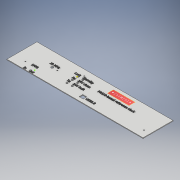
# Autodesk Inventor part: Panel
Saved by Autodesk Inventor 2018.2 (Build 222227000, 227)
## iProperties
Created: 2018-05-24
Part Number: Panel
Material: Generic
Document SubType Name: Modeling
Designer: ShifT
Density: 1 g/cm^3
Appearance: Default
Author: ShifT
Autodesk Inventor part; units mm, degrees
(part 1 of 3)
ref_plane "YZ Plane" through (0, 0, 0) normal (1, 0, 0) x (0, 1, 0)
ref_plane "XZ Plane" through (0, 0, 0) normal (0, 1, 0) x (-1, 0, 0)
ref_plane "XY Plane" through (0, 0, 0) normal (0, 0, 1) x (1, 0, 0)
sketch "Cutouts" plane through (0, 0, 0) normal (0, 0, 1) x (1, 0, 0)
  line L0 (-147.3514, 29.5026) -> (251.6486, 29.5026)
  line L1 (251.6486, 29.5026) -> (251.6486, -58.4974)
  line L2 (251.6486, -58.4974) -> (-147.3514, -58.4974)
  line L3 (-147.3514, -58.4974) -> (-147.3514, 29.5026)
  circle A0 centre (1, 0) radius 2.5548
  circle A1 centre (16.329, 0) radius 2.5548
  circle A2 centre (1, -15.329) radius 2.5548
  circle A3 centre (1, -30.6581) radius 2.5548
  circle A4 centre (16.329, -15.329) radius 2.5548
  circle A5 centre (16.329, -30.6581) radius 2.5548
  line L4 (53.6111, -37.1691) -> (65.6111, -37.1691)
  line L5 (65.6111, -37.1691) -> (65.6111, -47.8691)
  line L6 (65.6111, -47.8691) -> (53.6111, -47.8691)
  line L7 (53.6111, -47.8691) -> (53.6111, -37.1691)
  arc A6 (217.5748, -12.7276) -> (217.5951, -14.9758) centre (207.3252, -13.9442) ccw
  line L8 (217.6303, -12.7276) -> (218.5501, -12.7276)
  line L9 (218.5501, -12.7276) -> (218.5501, -14.9758)
  line L10 (218.5501, -14.9758) -> (217.5589, -14.9758)
  line L11 (207.3252, -13.9442) -> (219.4574, -13.9442) construction
  arc A7 (-61.8557, -10.0731) -> (-58.5401, -10.0731) centre (-60.1979, -12.8975) ccw
  line L12 (-61.8557, -10.0731) -> (-58.5401, -10.0731)
  arc A8 (-99.5904, -43.7211) -> (-96.2748, -43.7211) centre (-97.9326, -46.5455) ccw
  line L13 (-99.5904, -43.7211) -> (-96.2748, -43.7211)
  arc A9 (-80.2876, -43.5409) -> (-76.972, -43.5409) centre (-78.6298, -46.3653) ccw
  line L14 (-80.2876, -43.5409) -> (-76.972, -43.5409)
  circle A10 centre (9, 12) radius 1.5
  circle A11 centre (234, -38) radius 1.5
  circle A12 centre (-44.6116, -13.1835) radius 1.5
  circle A13 centre (-114.7272, -37.1581) radius 1.5
  point P0 (0, 0)
  dimension "d29" = 88
  dimension "d34" = 12
  dimension "d35" = 10.7
  dimension "d38" = 399
  dimension "d59" = 3.275
  dimension "d60" = 3.275
  dimension "d61" = 3.275
  constraints: 30 end point, 14 centre point, 8 point on circle, 5 horizontal, 5 parallel, 2 perpendicular, 2 point on line
  measures "d29" distance of L0.end L1.end
  measures "d34" distance of L4.start L4.end
  measures "d35" distance of L4.end L5.end
  measures "d38" distance of L0.start L0.end
  measures "d59" radius of A7
  measures "d60" radius of A9
  measures "d61" radius of A8
sketch "Text" plane through (0, 0, 0) normal (0, 0, 1) x (1, 0, 0)
  line L0 (-5.0504, -5.8552) -> (4.5125, -5.8552) construction
  line L1 (4.5125, -5.8552) -> (4.5125, -12.089) construction
  line L2 (4.5125, -12.089) -> (-5.0504, -12.089) construction
  line L3 (-5.0504, -12.089) -> (-5.0504, -5.8552) construction
  line L4 (-5.6331, -20.25) -> (3.6166, -20.25) construction
  line L5 (3.6166, -20.25) -> (3.6166, -26.4838) construction
  line L6 (3.6166, -26.4838) -> (-5.6331, -26.4838) construction
  line L7 (-5.6331, -26.4838) -> (-5.6331, -20.25) construction
  line L8 (11.6752, 9.4343) -> (42.3442, 9.4343) construction
  line L9 (42.3442, 9.4343) -> (42.3442, 1.2001) construction
  line L10 (42.3442, 1.2001) -> (11.6752, 1.2001) construction
  line L11 (11.6752, 1.2001) -> (11.6752, 9.4343) construction
  line L12 (11.9113, -5.446) -> (48.7686, -5.446) construction
  line L13 (48.7686, -5.446) -> (48.7686, -12.089) construction
  line L14 (48.7686, -12.089) -> (11.9113, -12.089) construction
  line L15 (11.9113, -12.089) -> (11.9113, -5.446) construction
  line L16 (12.7825, -20.3944) -> (46.5936, -20.3944) construction
  line L17 (46.5936, -20.3944) -> (46.5936, -27.0374) construction
  line L18 (46.5936, -27.0374) -> (12.7825, -27.0374) construction
  line L19 (12.7825, -27.0374) -> (12.7825, -20.3944) construction
  line L20 (-12.4705, 9.78) -> (4.6093, 9.78) construction
  line L21 (4.6093, 9.78) -> (4.6093, 1.0076) construction
  line L22 (4.6093, 1.0076) -> (-12.4705, 1.0076) construction
  line L23 (-12.4705, 1.0076) -> (-12.4705, 9.78) construction
  line L24 (-74.187, -1.4436) -> (-45.9479, -1.4436) construction
  line L25 (-45.9479, -1.4436) -> (-45.9479, -7.9351) construction
  line L26 (-45.9479, -7.9351) -> (-74.187, -7.9351) construction
  line L27 (-74.187, -7.9351) -> (-74.187, -1.4436) construction
  line L28 (-85.9199, -50.8606) -> (-71.5682, -50.8606) construction
  line L29 (-71.5682, -50.8606) -> (-71.5682, -58.0237) construction
  line L30 (-71.5682, -58.0237) -> (-85.9199, -58.0237) construction
  line L31 (-85.9199, -58.0237) -> (-85.9199, -50.8606) construction
  line L32 (-97.5821, -32.5156) -> (-80.0066, -32.5156) construction
  line L33 (-80.0066, -32.5156) -> (-80.0066, -38.9717) construction
  line L34 (-80.0066, -38.9717) -> (-97.5821, -38.9717) construction
  line L35 (-97.5821, -38.9717) -> (-97.5821, -32.5156) construction
  line L36 (69.2256, -39.9947) -> (96.6261, -39.9947) construction
  line L37 (96.6261, -39.9947) -> (96.6261, -46.4912) construction
  line L38 (96.6261, -46.4912) -> (69.2256, -46.4912) construction
  line L39 (69.2256, -46.4912) -> (69.2256, -39.9947) construction
  line L40 (86.2036, 20.2511) -> (149.6463, 20.2511) construction
  line L41 (149.6463, 20.2511) -> (149.6463, 2.3892) construction
  line L42 (149.6463, 2.3892) -> (86.2036, 2.3892) construction
  line L43 (86.2036, 2.3892) -> (86.2036, 20.2511) construction
  line L44 (67.8583, -2.9005) -> (181.6324, -2.9005) construction
  line L45 (181.6324, -2.9005) -> (181.6324, -16.7416) construction
  line L46 (181.6324, -16.7416) -> (67.8583, -16.7416) construction
  line L47 (67.8583, -16.7416) -> (67.8583, -2.9005) construction
  line L48 (-102.0131, -51.196) -> (-93.5064, -51.196) construction
  line L49 (-93.5064, -51.196) -> (-93.5064, -57.9236) construction
  line L50 (-93.5064, -57.9236) -> (-102.0131, -57.9236) construction
  line L51 (-102.0131, -57.9236) -> (-102.0131, -51.196) construction
  line L52 (-99.2695, -57.296) -> (-101.6324, -57.296)
  line L53 (-101.6324, -57.296) -> (-101.6324, -56.6731)
  line L54 (-101.6324, -56.6731) -> (-100.8563, -56.6731)
  line L55 (-100.8563, -56.6731) -> (-100.8563, -51.8188)
  line L56 (-100.8563, -51.8188) -> (-101.6324, -51.8188)
  line L57 (-101.6324, -51.8188) -> (-101.6324, -51.196)
  line L58 (-101.6324, -51.196) -> (-99.2695, -51.196)
  line L59 (-99.2695, -51.196) -> (-99.2695, -51.8188)
  line L60 (-99.2695, -51.8188) -> (-100.0456, -51.8188)
  line L61 (-100.0456, -51.8188) -> (-100.0456, -56.6731)
  line L62 (-100.0456, -56.6731) -> (-99.2695, -56.6731)
  line L63 (-99.2695, -56.6731) -> (-99.2695, -57.296)
  line L64 (-94.7316, -57.296) -> (-95.5028, -57.296)
  line L65 (-95.5028, -57.296) -> (-95.5028, -54.6859)
  spline S0 degree 2 poles (-95.5028, -54.6859) (-95.5028, -54.3696) (-95.5621, -53.8258) (-95.6511, -53.6627) knots 0 0 0 1 2 2 2
  spline S1 degree 2 poles (-95.6511, -53.6627) (-95.745, -53.4897) (-96.0811, -53.3216) (-96.3678, -53.3216) knots 0 0 0 1 2 2 2
  spline S2 degree 2 poles (-96.3678, -53.3216) (-96.6546, -53.3216) (-97.2626, -53.6281) (-97.5542, -53.8752) knots 0 0 0 1 2 2 2
  line L66 (-97.5542, -53.8752) -> (-97.5542, -57.296)
  line L67 (-97.5542, -57.296) -> (-98.3254, -57.296)
  line L68 (-98.3254, -57.296) -> (-98.3254, -52.7185)
  line L69 (-98.3254, -52.7185) -> (-97.5542, -52.7185)
  line L70 (-97.5542, -52.7185) -> (-97.5542, -53.2277)
  spline S3 degree 2 poles (-97.5542, -53.2277) (-97.2082, -52.9162) (-96.5409, -52.59) (-96.1652, -52.59) knots 0 0 0 1 2 2 2
  spline S4 degree 2 poles (-96.1652, -52.59) (-95.4929, -52.59) (-94.7316, -53.4798) (-94.7316, -54.3251) knots 0 0 0 1 2 2 2
  line L71 (-94.7316, -54.3251) -> (-94.7316, -57.296)
  line L72 (-70.2867, -7.6672) -> (-73.2626, -7.6672)
  line L73 (-73.2626, -7.6672) -> (-73.2626, -7.0443)
  line L74 (-73.2626, -7.0443) -> (-72.1553, -7.0443)
  line L75 (-72.1553, -7.0443) -> (-72.1553, -2.9563)
  line L76 (-72.1553, -2.9563) -> (-73.2626, -2.9563)
  line L77 (-73.2626, -2.9563) -> (-73.2626, -2.3977)
  spline S5 degree 2 poles (-73.2626, -2.3977) (-72.6348, -2.3977) (-72.0416, -2.0418) (-72.002, -1.5474) knots 0 0 0 1 2 2 2
  line L78 (-72.002, -1.5474) -> (-71.3693, -1.5474)
  line L79 (-71.3693, -1.5474) -> (-71.3693, -7.0443)
  line L80 (-71.3693, -7.0443) -> (-70.2867, -7.0443)
  line L81 (-70.2867, -7.0443) -> (-70.2867, -7.6672)
  spline S6 degree 2 poles (-65.3682, -4.6172) (-65.3682, -6.2584) (-66.3222, -7.7957) (-67.3158, -7.7957) knots 0 0 0 1 2 2 2
  spline S7 degree 2 poles (-67.3158, -7.7957) (-68.3243, -7.7957) (-69.2684, -6.2287) (-69.2684, -4.6221) knots 0 0 0 1 2 2 2
  spline S8 degree 2 poles (-69.2684, -4.6221) (-69.2684, -2.9711) (-68.3144, -1.4436) (-67.3158, -1.4436) knots 0 0 0 1 2 2 2
  spline S9 degree 2 poles (-67.3158, -1.4436) (-66.3123, -1.4436) (-65.3682, -3.0255) (-65.3682, -4.6172) knots 0 0 0 1 2 2 2
  spline S10 degree 2 poles (-66.4161, -6.4759) (-66.2975, -6.1743) (-66.1986, -5.245) (-66.1986, -4.6172) knots 0 0 0 1 2 2 2
  spline S11 degree 2 poles (-66.1986, -4.6172) (-66.1986, -3.9894) (-66.2975, -3.065) (-66.4211, -2.7536) knots 0 0 0 1 2 2 2
  spline S12 degree 2 poles (-66.4211, -2.7536) (-66.5447, -2.4422) (-66.9747, -2.1208) (-67.3158, -2.1208) knots 0 0 0 1 2 2 2
  spline S13 degree 2 poles (-67.3158, -2.1208) (-67.6569, -2.1208) (-68.0969, -2.4422) (-68.2254, -2.7635) knots 0 0 0 1 2 2 2
  spline S14 degree 2 poles (-68.2254, -2.7635) (-68.349, -3.0749) (-68.4379, -4.024) (-68.4379, -4.6221) knots 0 0 0 1 2 2 2
  spline S15 degree 2 poles (-68.4379, -4.6221) (-68.4379, -5.2648) (-68.3589, -6.1249) (-68.2303, -6.461) knots 0 0 0 1 2 2 2
  spline S16 degree 2 poles (-68.2303, -6.461) (-68.1117, -6.7774) (-67.6717, -7.1185) (-67.3158, -7.1185) knots 0 0 0 1 2 2 2
  spline S17 degree 2 poles (-67.3158, -7.1185) (-66.9797, -7.1185) (-66.5397, -6.7972) (-66.4161, -6.4759) knots 0 0 0 1 2 2 2
  line L82 (-56.5642, -7.6672) -> (-57.3749, -7.6672)
  line L83 (-57.3749, -7.6672) -> (-57.3749, -2.4125)
  line L84 (-57.3749, -2.4125) -> (-58.9666, -5.9865)
  line L85 (-58.9666, -5.9865) -> (-59.461, -5.9865)
  line L86 (-59.461, -5.9865) -> (-61.0379, -2.4125)
  line L87 (-61.0379, -2.4125) -> (-61.0379, -7.6672)
  line L88 (-61.0379, -7.6672) -> (-61.7942, -7.6672)
  line L89 (-61.7942, -7.6672) -> (-61.7942, -1.5672)
  line L90 (-61.7942, -1.5672) -> (-60.6869, -1.5672)
  line L91 (-60.6869, -1.5672) -> (-59.1644, -4.9632)
  line L92 (-59.1644, -4.9632) -> (-57.6913, -1.5672)
  line L93 (-57.6913, -1.5672) -> (-56.5642, -1.5672)
  line L94 (-56.5642, -1.5672) -> (-56.5642, -7.6672)
  line L95 (-50.8992, -7.6672) -> (-51.7099, -7.6672)
  line L96 (-51.7099, -7.6672) -> (-51.7099, -4.6815)
  line L97 (-51.7099, -4.6815) -> (-54.5177, -4.6815)
  line L98 (-54.5177, -4.6815) -> (-54.5177, -7.6672)
  line L99 (-54.5177, -7.6672) -> (-55.3284, -7.6672)
  line L100 (-55.3284, -7.6672) -> (-55.3284, -1.5672)
  line L101 (-55.3284, -1.5672) -> (-54.5177, -1.5672)
  line L102 (-54.5177, -1.5672) -> (-54.5177, -3.9597)
  line L103 (-54.5177, -3.9597) -> (-51.7099, -3.9597)
  line L104 (-51.7099, -3.9597) -> (-51.7099, -1.5672)
  line L105 (-51.7099, -1.5672) -> (-50.8992, -1.5672)
  line L106 (-50.8992, -1.5672) -> (-50.8992, -7.6672)
  line L107 (-46.7172, -7.6672) -> (-50.0786, -7.6672)
  line L108 (-50.0786, -7.6672) -> (-50.0786, -7.0938)
  line L109 (-50.0786, -7.0938) -> (-47.6861, -3.7225)
  line L110 (-47.6861, -3.7225) -> (-49.9798, -3.7225)
  line L111 (-49.9798, -3.7225) -> (-49.9798, -3.0897)
  line L112 (-49.9798, -3.0897) -> (-46.7617, -3.0897)
  line L113 (-46.7617, -3.0897) -> (-46.7617, -3.6384)
  line L114 (-46.7617, -3.6384) -> (-49.1641, -7.0196)
  line L115 (-49.1641, -7.0196) -> (-46.7172, -7.0196)
  line L116 (-46.7172, -7.0196) -> (-46.7172, -7.6672)
  line L117 (-8.3182, 3.4081) -> (-11.8526, 3.4081)
  line L118 (-11.8526, 3.4081) -> (-11.8526, 9.5081)
  line L119 (-11.8526, 9.5081) -> (-11.0419, 9.5081)
  line L120 (-11.0419, 9.5081) -> (-11.0419, 4.1298)
  line L121 (-11.0419, 4.1298) -> (-8.3182, 4.1298)
  line L122 (-8.3182, 4.1298) -> (-8.3182, 3.4081)
  spline S18 degree 2 poles (-3.978, 5.6968) (-3.978, 4.5401) (-5.0902, 3.2796) (-6.0195, 3.2796) knots 0 0 0 1 2 2 2
  spline S19 degree 2 poles (-6.0195, 3.2796) (-6.9736, 3.2796) (-8.066, 4.5797) (-8.066, 5.6968) knots 0 0 0 1 2 2 2
  spline S20 degree 2 poles (-8.066, 5.6968) (-8.066, 6.8437) (-6.939, 8.1141) (-6.0195, 8.1141) knots 0 0 0 1 2 2 2
  spline S21 degree 2 poles (-6.0195, 8.1141) (-5.0902, 8.1141) (-3.978, 6.8486) (-3.978, 5.6968) knots 0 0 0 1 2 2 2
  spline S22 degree 2 poles (-4.7738, 5.6968) (-4.7738, 6.5866) (-5.4214, 7.4517) (-6.0195, 7.4517) knots 0 0 0 1 2 2 2
  spline S23 degree 2 poles (-6.0195, 7.4517) (-6.6177, 7.4517) (-7.2702, 6.5866) (-7.2702, 5.6968) knots 0 0 0 1 2 2 2
  spline S24 degree 2 poles (-7.2702, 5.6968) (-7.2702, 4.8318) (-6.6177, 3.942) (-6.0195, 3.942) knots 0 0 0 1 2 2 2
  spline S25 degree 2 poles (-6.0195, 3.942) (-5.4263, 3.942) (-4.7738, 4.8169) (-4.7738, 5.6968) knots 0 0 0 1 2 2 2
  spline S26 degree 2 poles (-1.3679, 3.3043) (-1.8425, 3.3043) (-2.6284, 3.596) (-2.9102, 3.8925) knots 0 0 0 1 2 2 2
  spline S27 degree 2 poles (-2.9102, 3.8925) (-3.192, 4.1842) (-3.5034, 5.0839) (-3.5034, 5.687) knots 0 0 0 1 2 2 2
  spline S28 degree 2 poles (-3.5034, 5.687) (-3.5034, 6.29) (-3.1821, 7.1699) (-2.9102, 7.4665) knots 0 0 0 1 2 2 2
  spline S29 degree 2 poles (-2.9102, 7.4665) (-2.6383, 7.7681) (-1.8326, 8.0894) (-1.3679, 8.0894) knots 0 0 0 1 2 2 2
  spline S30 degree 2 poles (-1.3679, 8.0894) (-0.9922, 8.0894) (-0.2903, 7.8768) (-0.0184, 7.7384) knots 0 0 0 1 2 2 2
  line L123 (-0.0184, 7.7384) -> (-0.0184, 6.8733)
  line L124 (-0.0184, 6.8733) -> (-0.0629, 6.8733)
  spline S31 degree 2 poles (-0.0629, 6.8733) (-0.1469, 6.9425) (-0.404, 7.1205) (-0.5869, 7.2144) knots 0 0 0 1 2 2 2
  spline S32 degree 2 poles (-0.5869, 7.2144) (-0.75, 7.2935) (-1.185, 7.4171) (-1.3827, 7.4171) knots 0 0 0 1 2 2 2
  spline S33 degree 2 poles (-1.3827, 7.4171) (-1.9809, 7.4171) (-2.7075, 6.5125) (-2.7075, 5.687) knots 0 0 0 1 2 2 2
  spline S34 degree 2 poles (-2.7075, 5.687) (-2.7075, 4.8812) (-2.0056, 3.9766) (-1.3827, 3.9766) knots 0 0 0 1 2 2 2
  spline S35 degree 2 poles (-1.3827, 3.9766) (-1.0071, 3.9766) (-0.3249, 4.288) (-0.0629, 4.5302) knots 0 0 0 1 2 2 2
  line L125 (-0.0629, 4.5302) -> (-0.0184, 4.5302)
  line L126 (-0.0184, 4.5302) -> (-0.0184, 3.6652)
  spline S36 degree 2 poles (-0.0184, 3.6652) (-0.1321, 3.6108) (-0.4781, 3.4575) (-0.6165, 3.4229) knots 0 0 0 1 2 2 2
  spline S37 degree 2 poles (-0.6165, 3.4229) (-0.8143, 3.3636) (-1.1257, 3.3043) (-1.3679, 3.3043) knots 0 0 0 1 2 2 2
  line L127 (4.475, 3.4081) -> (3.4617, 3.4081)
  line L128 (3.4617, 3.4081) -> (1.7612, 5.6177)
  line L129 (1.7612, 5.6177) -> (1.4547, 5.3212)
  line L130 (1.4547, 5.3212) -> (1.4547, 3.4081)
  line L131 (1.4547, 3.4081) -> (0.6835, 3.4081)
  line L132 (0.6835, 3.4081) -> (0.6835, 9.78)
  line L133 (0.6835, 9.78) -> (1.4547, 9.78)
  line L134 (1.4547, 9.78) -> (1.4547, 6.0528)
  line L135 (1.4547, 6.0528) -> (3.2639, 7.9856)
  line L136 (3.2639, 7.9856) -> (4.2229, 7.9856)
  line L137 (4.2229, 7.9856) -> (2.3445, 6.0725)
  line L138 (2.3445, 6.0725) -> (4.475, 3.4081)
  spline S38 degree 2 poles (-80.9865, -51.6861) (-80.6405, -52.0914) (-80.2549, -53.2778) (-80.2549, -54.0391) knots 0 0 0 1 2 2 2
  spline S39 degree 2 poles (-80.2549, -54.0391) (-80.2549, -54.7806) (-80.6306, -55.9818) (-80.9865, -56.3871) knots 0 0 0 1 2 2 2
  spline S40 degree 2 poles (-80.9865, -56.3871) (-81.3622, -56.8123) (-82.3558, -57.2176) (-82.954, -57.2176) knots 0 0 0 1 2 2 2
  spline S41 degree 2 poles (-82.954, -57.2176) (-83.5719, -57.2176) (-84.5605, -56.7974) (-84.9214, -56.3871) knots 0 0 0 1 2 2 2
  spline S42 degree 2 poles (-84.9214, -56.3871) (-85.2724, -55.9818) (-85.648, -54.7905) (-85.648, -54.0391) knots 0 0 0 1 2 2 2
  spline S43 degree 2 poles (-85.648, -54.0391) (-85.648, -53.2729) (-85.2674, -52.1063) (-84.9164, -51.6861) knots 0 0 0 1 2 2 2
  spline S44 degree 2 poles (-84.9164, -51.6861) (-84.5605, -51.2807) (-83.5669, -50.8606) (-82.954, -50.8606) knots 0 0 0 1 2 2 2
  spline S45 degree 2 poles (-82.954, -50.8606) (-82.3311, -50.8606) (-81.3326, -51.2956) (-80.9865, -51.6861) knots 0 0 0 1 2 2 2
  spline S46 degree 2 poles (-81.1002, -54.0391) (-81.1002, -53.436) (-81.3622, -52.5017) (-81.5995, -52.1952) knots 0 0 0 1 2 2 2
  spline S47 degree 2 poles (-81.5995, -52.1952) (-81.8417, -51.8789) (-82.5239, -51.5625) (-82.949, -51.5625) knots 0 0 0 1 2 2 2
  spline S48 degree 2 poles (-82.949, -51.5625) (-83.389, -51.5625) (-84.0514, -51.869) (-84.3035, -52.1952) knots 0 0 0 1 2 2 2
  spline S49 degree 2 poles (-84.3035, -52.1952) (-84.5457, -52.5067) (-84.8027, -53.4459) (-84.8027, -54.0391) knots 0 0 0 1 2 2 2
  spline S50 degree 2 poles (-84.8027, -54.0391) (-84.8027, -55.2403) (-83.7943, -56.5157) (-82.949, -56.5157) knots 0 0 0 1 2 2 2
  spline S51 degree 2 poles (-82.949, -56.5157) (-82.1037, -56.5157) (-81.1002, -55.2403) (-81.1002, -54.0391) knots 0 0 0 1 2 2 2
  line L139 (-75.8653, -57.0891) -> (-76.6365, -57.0891)
  line L140 (-76.6365, -57.0891) -> (-76.6365, -56.5849)
  spline S52 degree 2 poles (-76.6365, -56.5849) (-76.9924, -56.8963) (-77.6301, -57.2176) (-78.0255, -57.2176) knots 0 0 0 1 2 2 2
  spline S53 degree 2 poles (-78.0255, -57.2176) (-78.3221, -57.2176) (-78.851, -57.0199) (-79.0438, -56.8073) knots 0 0 0 1 2 2 2
  spline S54 degree 2 poles (-79.0438, -56.8073) (-79.2416, -56.5948) (-79.4591, -55.9472) (-79.4591, -55.4825) knots 0 0 0 1 2 2 2
  line L141 (-79.4591, -55.4825) -> (-79.4591, -52.5116)
  line L142 (-79.4591, -52.5116) -> (-78.6879, -52.5116)
  line L143 (-78.6879, -52.5116) -> (-78.6879, -55.1217)
  spline S55 degree 2 poles (-78.6879, -55.1217) (-78.6879, -55.4875) (-78.6335, -55.967) (-78.5396, -56.1449) knots 0 0 0 1 2 2 2
  spline S56 degree 2 poles (-78.5396, -56.1449) (-78.4457, -56.3229) (-78.1244, -56.486) (-77.8228, -56.486) knots 0 0 0 1 2 2 2
  spline S57 degree 2 poles (-77.8228, -56.486) (-77.5411, -56.486) (-76.9034, -56.1647) (-76.6365, -55.9324) knots 0 0 0 1 2 2 2
  line L144 (-76.6365, -55.9324) -> (-76.6365, -52.5116)
  line L145 (-76.6365, -52.5116) -> (-75.8653, -52.5116)
  line L146 (-75.8653, -52.5116) -> (-75.8653, -57.0891)
  spline S58 degree 2 poles (-73.364, -57.1781) (-73.9918, -57.1781) (-74.6987, -56.4613) (-74.6987, -55.6852) knots 0 0 0 1 2 2 2
  line L147 (-74.6987, -55.6852) -> (-74.6987, -53.1493)
  line L148 (-74.6987, -53.1493) -> (-75.2177, -53.1493)
  line L149 (-75.2177, -53.1493) -> (-75.2177, -52.5116)
  line L150 (-75.2177, -52.5116) -> (-74.6987, -52.5116)
  line L151 (-74.6987, -52.5116) -> (-74.6987, -51.1967)
  line L152 (-74.6987, -51.1967) -> (-73.9275, -51.1967)
  line L153 (-73.9275, -51.1967) -> (-73.9275, -52.5116)
  line L154 (-73.9275, -52.5116) -> (-72.5088, -52.5116)
  line L155 (-72.5088, -52.5116) -> (-72.5088, -53.1493)
  line L156 (-72.5088, -53.1493) -> (-73.9275, -53.1493)
  line L157 (-73.9275, -53.1493) -> (-73.9275, -55.3293)
  spline S59 degree 2 poles (-73.9275, -55.3293) (-73.9275, -55.6753) (-73.9028, -56.0559) (-73.8188, -56.2191) knots 0 0 0 1 2 2 2
  spline S60 degree 2 poles (-73.8188, -56.2191) (-73.7496, -56.3624) (-73.4382, -56.5058) (-73.1712, -56.5058) knots 0 0 0 1 2 2 2
  spline S61 degree 2 poles (-73.1712, -56.5058) (-72.9834, -56.5058) (-72.6324, -56.3921) (-72.5533, -56.3575) knots 0 0 0 1 2 2 2
  line L158 (-72.5533, -56.3575) -> (-72.5088, -56.3575)
  line L159 (-72.5088, -56.3575) -> (-72.5088, -57.0495)
  spline S62 degree 2 poles (-72.5088, -57.0495) (-72.7263, -57.1089) (-73.1712, -57.1781) (-73.364, -57.1781) knots 0 0 0 1 2 2 2
  line L160 (-93.6819, -38.7244) -> (-96.6577, -38.7244)
  line L161 (-96.6577, -38.7244) -> (-96.6577, -38.1015)
  line L162 (-96.6577, -38.1015) -> (-95.5504, -38.1015)
  line L163 (-95.5504, -38.1015) -> (-95.5504, -34.0134)
  line L164 (-95.5504, -34.0134) -> (-96.6577, -34.0134)
  line L165 (-96.6577, -34.0134) -> (-96.6577, -33.4548)
  spline S63 degree 2 poles (-96.6577, -33.4548) (-96.0299, -33.4548) (-95.4367, -33.0989) (-95.3972, -32.6046) knots 0 0 0 1 2 2 2
  line L166 (-95.3972, -32.6046) -> (-94.7644, -32.6046)
  line L167 (-94.7644, -32.6046) -> (-94.7644, -38.1015)
  line L168 (-94.7644, -38.1015) -> (-93.6819, -38.1015)
  line L169 (-93.6819, -38.1015) -> (-93.6819, -38.7244)
  spline S64 degree 2 poles (-88.531, -34.4632) (-88.531, -34.8587) (-88.8127, -35.5705) (-89.0648, -35.8177) knots 0 0 0 1 2 2 2
  spline S65 degree 2 poles (-89.0648, -35.8177) (-89.3812, -36.1291) (-90.2364, -36.4504) (-90.8889, -36.4504) knots 0 0 0 1 2 2 2
  line L170 (-90.8889, -36.4504) -> (-91.576, -36.4504)
  line L171 (-91.576, -36.4504) -> (-91.576, -38.7244)
  line L172 (-91.576, -38.7244) -> (-92.3867, -38.7244)
  line L173 (-92.3867, -38.7244) -> (-92.3867, -32.6244)
  line L174 (-92.3867, -32.6244) -> (-90.8543, -32.6244)
  spline S66 degree 2 poles (-90.8543, -32.6244) (-90.3105, -32.6244) (-89.5493, -32.8023) (-89.2576, -33.005) knots 0 0 0 1 2 2 2
  spline S67 degree 2 poles (-89.2576, -33.005) (-88.9165, -33.2373) (-88.531, -33.9541) (-88.531, -34.4632) knots 0 0 0 1 2 2 2
  spline S68 degree 2 poles (-89.3763, -34.488) (-89.3763, -34.1716) (-89.5938, -33.7069) (-89.8162, -33.5586) knots 0 0 0 1 2 2 2
  spline S69 degree 2 poles (-89.8162, -33.5586) (-90.009, -33.4301) (-90.5231, -33.3263) (-90.9037, -33.3263) knots 0 0 0 1 2 2 2
  line L175 (-90.9037, -33.3263) -> (-91.576, -33.3263)
  line L176 (-91.576, -33.3263) -> (-91.576, -35.7584)
  line L177 (-91.576, -35.7584) -> (-91.0224, -35.7584)
  spline S70 degree 2 poles (-91.0224, -35.7584) (-90.528, -35.7584) (-89.92, -35.6002) (-89.7223, -35.3926) knots 0 0 0 1 2 2 2
  spline S71 degree 2 poles (-89.7223, -35.3926) (-89.5394, -35.2097) (-89.3763, -34.7796) (-89.3763, -34.488) knots 0 0 0 1 2 2 2
  spline S72 degree 2 poles (-83.9041, -34.4632) (-83.9041, -34.8587) (-84.1858, -35.5705) (-84.4379, -35.8177) knots 0 0 0 1 2 2 2
  spline S73 degree 2 poles (-84.4379, -35.8177) (-84.7543, -36.1291) (-85.6095, -36.4504) (-86.262, -36.4504) knots 0 0 0 1 2 2 2
  line L178 (-86.262, -36.4504) -> (-86.9491, -36.4504)
  line L179 (-86.9491, -36.4504) -> (-86.9491, -38.7244)
  line L180 (-86.9491, -38.7244) -> (-87.7598, -38.7244)
  line L181 (-87.7598, -38.7244) -> (-87.7598, -32.6244)
  line L182 (-87.7598, -32.6244) -> (-86.2274, -32.6244)
  spline S74 degree 2 poles (-86.2274, -32.6244) (-85.6836, -32.6244) (-84.9224, -32.8023) (-84.6307, -33.005) knots 0 0 0 1 2 2 2
  spline S75 degree 2 poles (-84.6307, -33.005) (-84.2896, -33.2373) (-83.9041, -33.9541) (-83.9041, -34.4632) knots 0 0 0 1 2 2 2
  spline S76 degree 2 poles (-84.7494, -34.488) (-84.7494, -34.1716) (-84.9669, -33.7069) (-85.1893, -33.5586) knots 0 0 0 1 2 2 2
  spline S77 degree 2 poles (-85.1893, -33.5586) (-85.3821, -33.4301) (-85.8962, -33.3263) (-86.2768, -33.3263) knots 0 0 0 1 2 2 2
  line L183 (-86.2768, -33.3263) -> (-86.9491, -33.3263)
  line L184 (-86.9491, -33.3263) -> (-86.9491, -35.7584)
  line L185 (-86.9491, -35.7584) -> (-86.3955, -35.7584)
  spline S78 degree 2 poles (-86.3955, -35.7584) (-85.9011, -35.7584) (-85.2931, -35.6002) (-85.0954, -35.3926) knots 0 0 0 1 2 2 2
  spline S79 degree 2 poles (-85.0954, -35.3926) (-84.9125, -35.2097) (-84.7494, -34.7796) (-84.7494, -34.488) knots 0 0 0 1 2 2 2
  spline S80 degree 2 poles (-81.4324, -38.8331) (-82.0948, -38.8331) (-83.0242, -38.5563) (-83.4344, -38.3585) knots 0 0 0 1 2 2 2
  line L186 (-83.4344, -38.3585) -> (-83.4344, -37.3402)
  line L187 (-83.4344, -37.3402) -> (-83.3751, -37.3402)
  spline S81 degree 2 poles (-83.3751, -37.3402) (-82.9747, -37.7159) (-81.9614, -38.1312) (-81.4917, -38.1312) knots 0 0 0 1 2 2 2
  spline S82 degree 2 poles (-81.4917, -38.1312) (-80.8195, -38.1312) (-80.1323, -37.5726) (-80.1323, -37.1128) knots 0 0 0 1 2 2 2
  spline S83 degree 2 poles (-80.1323, -37.1128) (-80.1323, -36.747) (-80.4932, -36.2923) (-80.8837, -36.1786) knots 0 0 0 1 2 2 2
  spline S84 degree 2 poles (-80.8837, -36.1786) (-81.1655, -36.0995) (-81.6351, -35.9907) (-81.9861, -35.9017) knots 0 0 0 1 2 2 2
  spline S85 degree 2 poles (-81.9861, -35.9017) (-82.3024, -35.8177) (-82.8017, -35.5656) (-82.9945, -35.3629) knots 0 0 0 1 2 2 2
  spline S86 degree 2 poles (-82.9945, -35.3629) (-83.1823, -35.1603) (-83.39, -34.6165) (-83.39, -34.2606) knots 0 0 0 1 2 2 2
  spline S87 degree 2 poles (-83.39, -34.2606) (-83.39, -33.5191) (-82.2332, -32.5156) (-81.3385, -32.5156) knots 0 0 0 1 2 2 2
  spline S88 degree 2 poles (-81.3385, -32.5156) (-80.8244, -32.5156) (-79.9148, -32.7183) (-79.5243, -32.9111) knots 0 0 0 1 2 2 2
  line L188 (-79.5243, -32.9111) -> (-79.5243, -33.8799)
  line L189 (-79.5243, -33.8799) -> (-79.5836, -33.8799)
  spline S89 degree 2 poles (-79.5836, -33.8799) (-79.8753, -33.613) (-80.7849, -33.2175) (-81.2841, -33.2175) knots 0 0 0 1 2 2 2
  spline S90 degree 2 poles (-81.2841, -33.2175) (-81.8477, -33.2175) (-82.5447, -33.7465) (-82.5447, -34.1765) knots 0 0 0 1 2 2 2
  spline S91 degree 2 poles (-82.5447, -34.1765) (-82.5447, -34.5621) (-82.1344, -35.0218) (-81.7488, -35.1256) knots 0 0 0 1 2 2 2
  spline S92 degree 2 poles (-81.7488, -35.1256) (-81.4917, -35.1949) (-80.7453, -35.3728) (-80.4981, -35.447) knots 0 0 0 1 2 2 2
  spline S93 degree 2 poles (-80.4981, -35.447) (-79.8703, -35.6397) (-79.287, -36.4158) (-79.287, -36.9843) knots 0 0 0 1 2 2 2
  spline S94 degree 2 poles (-79.287, -36.9843) (-79.287, -37.3452) (-79.5787, -38.0372) (-79.8407, -38.2795) knots 0 0 0 1 2 2 2
  spline S95 degree 2 poles (-79.8407, -38.2795) (-80.1323, -38.5464) (-80.8738, -38.8331) (-81.4324, -38.8331) knots 0 0 0 1 2 2 2
  spline S96 degree 2 poles (71.974, -46.3517) (71.4352, -46.3517) (70.6344, -46.07) (70.3527, -45.7882) knots 0 0 0 1 2 2 2
  spline S97 degree 2 poles (70.3527, -45.7882) (70.0313, -45.4718) (69.7693, -44.5821) (69.7693, -43.9295) knots 0 0 0 1 2 2 2
  line L190 (69.7693, -43.9295) -> (69.7693, -40.1232)
  line L191 (69.7693, -40.1232) -> (70.58, -40.1232)
  line L192 (70.58, -40.1232) -> (70.58, -43.9295)
  spline S98 degree 2 poles (70.58, -43.9295) (70.58, -44.3547) (70.6888, -44.9281) (70.842, -45.1604) knots 0 0 0 1 2 2 2
  spline S99 degree 2 poles (70.842, -45.1604) (71.0052, -45.4076) (71.5687, -45.6597) (71.974, -45.6597) knots 0 0 0 1 2 2 2
  spline S100 degree 2 poles (71.974, -45.6597) (72.3547, -45.6597) (72.9479, -45.4076) (73.111, -45.1604) knots 0 0 0 1 2 2 2
  spline S101 degree 2 poles (73.111, -45.1604) (73.2642, -44.9281) (73.373, -44.3596) (73.373, -43.9493) knots 0 0 0 1 2 2 2
  line L193 (73.373, -43.9493) -> (73.373, -40.1232)
  line L194 (73.373, -40.1232) -> (74.1837, -40.1232)
  line L195 (74.1837, -40.1232) -> (74.1837, -43.9295)
  spline S102 degree 2 poles (74.1837, -43.9295) (74.1837, -44.5672) (73.9266, -45.4768) (73.6004, -45.7882) knots 0 0 0 1 2 2 2
  spline S103 degree 2 poles (73.6004, -45.7882) (73.3087, -46.0749) (72.5376, -46.3517) (71.974, -46.3517) knots 0 0 0 1 2 2 2
  spline S104 degree 2 poles (77.0458, -46.332) (76.3834, -46.332) (75.4541, -46.0552) (75.0438, -45.8574) knots 0 0 0 1 2 2 2
  line L196 (75.0438, -45.8574) -> (75.0438, -44.8391)
  line L197 (75.0438, -44.8391) -> (75.1031, -44.8391)
  spline S105 degree 2 poles (75.1031, -44.8391) (75.5035, -45.2148) (76.5169, -45.63) (76.9865, -45.63) knots 0 0 0 1 2 2 2
  spline S106 degree 2 poles (76.9865, -45.63) (77.6588, -45.63) (78.3459, -45.0714) (78.3459, -44.6117) knots 0 0 0 1 2 2 2
  spline S107 degree 2 poles (78.3459, -44.6117) (78.3459, -44.2459) (77.9851, -43.7911) (77.5945, -43.6774) knots 0 0 0 1 2 2 2
  spline S108 degree 2 poles (77.5945, -43.6774) (77.3128, -43.5983) (76.8432, -43.4896) (76.4922, -43.4006) knots 0 0 0 1 2 2 2
  spline S109 degree 2 poles (76.4922, -43.4006) (76.1758, -43.3166) (75.6766, -43.0645) (75.4838, -42.8618) knots 0 0 0 1 2 2 2
  spline S110 degree 2 poles (75.4838, -42.8618) (75.2959, -42.6591) (75.0883, -42.1154) (75.0883, -41.7594) knots 0 0 0 1 2 2 2
  spline S111 degree 2 poles (75.0883, -41.7594) (75.0883, -41.018) (76.245, -40.0145) (77.1398, -40.0145) knots 0 0 0 1 2 2 2
  spline S112 degree 2 poles (77.1398, -40.0145) (77.6539, -40.0145) (78.5634, -40.2171) (78.9539, -40.4099) knots 0 0 0 1 2 2 2
  line L198 (78.9539, -40.4099) -> (78.9539, -41.3788)
  line L199 (78.9539, -41.3788) -> (78.8946, -41.3788)
  spline S113 degree 2 poles (78.8946, -41.3788) (78.603, -41.1119) (77.6934, -40.7164) (77.1941, -40.7164) knots 0 0 0 1 2 2 2
  spline S114 degree 2 poles (77.1941, -40.7164) (76.6306, -40.7164) (75.9336, -41.2453) (75.9336, -41.6754) knots 0 0 0 1 2 2 2
  spline S115 degree 2 poles (75.9336, -41.6754) (75.9336, -42.061) (76.3439, -42.5207) (76.7295, -42.6245) knots 0 0 0 1 2 2 2
  spline S116 degree 2 poles (76.7295, -42.6245) (76.9865, -42.6937) (77.733, -42.8717) (77.9801, -42.9458) knots 0 0 0 1 2 2 2
  spline S117 degree 2 poles (77.9801, -42.9458) (78.6079, -43.1386) (79.1912, -43.9147) (79.1912, -44.4832) knots 0 0 0 1 2 2 2
  spline S118 degree 2 poles (79.1912, -44.4832) (79.1912, -44.8441) (78.8996, -45.5361) (78.6376, -45.7783) knots 0 0 0 1 2 2 2
  spline S119 degree 2 poles (78.6376, -45.7783) (78.3459, -46.0453) (77.6044, -46.332) (77.0458, -46.332) knots 0 0 0 1 2 2 2
  spline S120 degree 2 poles (84.1543, -44.3497) (84.1543, -44.8045) (83.8082, -45.5015) (83.5215, -45.7289) knots 0 0 0 1 2 2 2
  spline S121 degree 2 poles (83.5215, -45.7289) (83.1755, -45.9958) (82.3895, -46.2232) (81.7667, -46.2232) knots 0 0 0 1 2 2 2
  line L200 (81.7667, -46.2232) -> (80.0168, -46.2232)
  line L201 (80.0168, -46.2232) -> (80.0168, -40.1232)
  line L202 (80.0168, -40.1232) -> (81.6332, -40.1232)
  spline S122 degree 2 poles (81.6332, -40.1232) (82.2857, -40.1232) (82.9382, -40.2073) (83.2348, -40.3704) knots 0 0 0 1 2 2 2
  spline S123 degree 2 poles (83.2348, -40.3704) (83.566, -40.5434) (83.8676, -41.1119) (83.8676, -41.4975) knots 0 0 0 1 2 2 2
  spline S124 degree 2 poles (83.8676, -41.4975) (83.8676, -41.9275) (83.4128, -42.6097) (83.0124, -42.8025) knots 0 0 0 1 2 2 2
  line L203 (83.0124, -42.8025) -> (83.0124, -42.8321)
  spline S125 degree 2 poles (83.0124, -42.8321) (83.5561, -42.9804) (84.1543, -43.7664) (84.1543, -44.3497) knots 0 0 0 1 2 2 2
  spline S126 degree 2 poles (83.309, -44.3843) (83.309, -44.0383) (83.1112, -43.5934) (82.8146, -43.4352) knots 0 0 0 1 2 2 2
  spline S127 degree 2 poles (82.8146, -43.4352) (82.6219, -43.3364) (82.1671, -43.277) (81.7469, -43.277) knots 0 0 0 1 2 2 2
  line L204 (81.7469, -43.277) -> (80.8274, -43.277)
  line L205 (80.8274, -43.277) -> (80.8274, -45.5312)
  line L206 (80.8274, -45.5312) -> (81.4849, -45.5312)
  spline S128 degree 2 poles (81.4849, -45.5312) (82.0188, -45.5312) (82.6317, -45.4323) (82.869, -45.2741) knots 0 0 0 1 2 2 2
  spline S129 degree 2 poles (82.869, -45.2741) (83.0964, -45.111) (83.309, -44.7056) (83.309, -44.3843) knots 0 0 0 1 2 2 2
  spline S130 degree 2 poles (83.0223, -41.6111) (83.0223, -41.3936) (82.874, -41.0674) (82.7108, -40.9735) knots 0 0 0 1 2 2 2
  spline S131 degree 2 poles (82.7108, -40.9735) (82.5131, -40.8647) (82.0336, -40.8153) (81.6035, -40.8153) knots 0 0 0 1 2 2 2
  line L207 (81.6035, -40.8153) -> (80.8274, -40.8153)
  line L208 (80.8274, -40.8153) -> (80.8274, -42.5998)
  line L209 (80.8274, -42.5998) -> (81.7469, -42.5998)
  spline S132 degree 2 poles (81.7469, -42.5998) (82.1275, -42.5998) (82.4884, -42.5207) (82.6812, -42.3971) knots 0 0 0 1 2 2 2
  spline S133 degree 2 poles (82.6812, -42.3971) (82.869, -42.2785) (83.0223, -41.8979) (83.0223, -41.6111) knots 0 0 0 1 2 2 2
  line L210 (88.5488, -46.2232) -> (84.787, -46.2232)
  line L211 (84.787, -46.2232) -> (84.787, -45.3582)
  spline S134 degree 2 poles (84.787, -45.3582) (85.1924, -44.9775) (85.9141, -44.2706) (86.2601, -43.89) knots 0 0 0 1 2 2 2
  spline S135 degree 2 poles (86.2601, -43.89) (86.9571, -43.1238) (87.4663, -42.2043) (87.4663, -41.715) knots 0 0 0 1 2 2 2
  spline S136 degree 2 poles (87.4663, -41.715) (87.4663, -41.4579) (87.3081, -41.0723) (87.1647, -40.9488) knots 0 0 0 1 2 2 2
  spline S137 degree 2 poles (87.1647, -40.9488) (87.0214, -40.8252) (86.6457, -40.7016) (86.4183, -40.7016) knots 0 0 0 1 2 2 2
  spline S138 degree 2 poles (86.4183, -40.7016) (86.2008, -40.7016) (85.7559, -40.8103) (85.5532, -40.8944) knots 0 0 0 1 2 2 2
  spline S139 degree 2 poles (85.5532, -40.8944) (85.3802, -40.9636) (85.0589, -41.1613) (84.96, -41.2305) knots 0 0 0 1 2 2 2
  line L212 (84.96, -41.2305) -> (84.9155, -41.2305)
  line L213 (84.9155, -41.2305) -> (84.9155, -40.3605)
  spline S140 degree 2 poles (84.9155, -40.3605) (85.1676, -40.2369) (86.0723, -39.9947) (86.4776, -39.9947) knots 0 0 0 1 2 2 2
  spline S141 degree 2 poles (86.4776, -39.9947) (87.3328, -39.9947) (88.2967, -40.8993) (88.2967, -41.6705) knots 0 0 0 1 2 2 2
  spline S142 degree 2 poles (88.2967, -41.6705) (88.2967, -42.0313) (88.1287, -42.6344) (87.9804, -42.8915) knots 0 0 0 1 2 2 2
  spline S143 degree 2 poles (87.9804, -42.8915) (87.8321, -43.1584) (87.402, -43.6824) (87.1647, -43.9345) knots 0 0 0 1 2 2 2
  spline S144 degree 2 poles (87.1647, -43.9345) (86.7792, -44.3547) (85.835, -45.2543) (85.5532, -45.5163) knots 0 0 0 1 2 2 2
  line L214 (85.5532, -45.5163) -> (88.5488, -45.5163)
  line L215 (88.5488, -45.5163) -> (88.5488, -46.2232)
  line L216 (90.6745, -46.2232) -> (89.6957, -46.2232)
  line L217 (89.6957, -46.2232) -> (89.6957, -45.0566)
  line L218 (89.6957, -45.0566) -> (90.6745, -45.0566)
  line L219 (90.6745, -45.0566) -> (90.6745, -46.2232)
  spline S145 degree 2 poles (95.7018, -43.1732) (95.7018, -44.8144) (94.7477, -46.3517) (93.7541, -46.3517) knots 0 0 0 1 2 2 2
  spline S146 degree 2 poles (93.7541, -46.3517) (92.7457, -46.3517) (91.8015, -44.7847) (91.8015, -43.1782) knots 0 0 0 1 2 2 2
  spline S147 degree 2 poles (91.8015, -43.1782) (91.8015, -41.5271) (92.7556, -39.9996) (93.7541, -39.9996) knots 0 0 0 1 2 2 2
  spline S148 degree 2 poles (93.7541, -39.9996) (94.7576, -39.9996) (95.7018, -41.5815) (95.7018, -43.1732) knots 0 0 0 1 2 2 2
  spline S149 degree 2 poles (94.6538, -45.0319) (94.7724, -44.7304) (94.8713, -43.801) (94.8713, -43.1732) knots 0 0 0 1 2 2 2
  spline S150 degree 2 poles (94.8713, -43.1732) (94.8713, -42.5454) (94.7724, -41.621) (94.6488, -41.3096) knots 0 0 0 1 2 2 2
  spline S151 degree 2 poles (94.6488, -41.3096) (94.5253, -40.9982) (94.0952, -40.6769) (93.7541, -40.6769) knots 0 0 0 1 2 2 2
  spline S152 degree 2 poles (93.7541, -40.6769) (93.413, -40.6769) (92.9731, -40.9982) (92.8445, -41.3195) knots 0 0 0 1 2 2 2
  spline S153 degree 2 poles (92.8445, -41.3195) (92.721, -41.6309) (92.632, -42.58) (92.632, -43.1782) knots 0 0 0 1 2 2 2
  spline S154 degree 2 poles (92.632, -43.1782) (92.632, -43.8208) (92.7111, -44.6809) (92.8396, -45.0171) knots 0 0 0 1 2 2 2
  spline S155 degree 2 poles (92.8396, -45.0171) (92.9582, -45.3334) (93.3982, -45.6745) (93.7541, -45.6745) knots 0 0 0 1 2 2 2
  spline S156 degree 2 poles (93.7541, -45.6745) (94.0903, -45.6745) (94.5302, -45.3532) (94.6538, -45.0319) knots 0 0 0 1 2 2 2
  spline S157 degree 2 poles (13.9936, 2.9537) (13.3312, 2.9537) (12.4019, 3.2305) (11.9916, 3.4283) knots 0 0 0 1 2 2 2
  line L220 (11.9916, 3.4283) -> (11.9916, 4.4466)
  line L221 (11.9916, 4.4466) -> (12.0509, 4.4466)
  spline S158 degree 2 poles (12.0509, 4.4466) (12.4513, 4.0709) (13.4647, 3.6557) (13.9343, 3.6557) knots 0 0 0 1 2 2 2
  spline S159 degree 2 poles (13.9343, 3.6557) (14.6066, 3.6557) (15.2937, 4.2142) (15.2937, 4.674) knots 0 0 0 1 2 2 2
  spline S160 degree 2 poles (15.2937, 4.674) (15.2937, 5.0398) (14.9328, 5.4946) (14.5423, 5.6082) knots 0 0 0 1 2 2 2
  spline S161 degree 2 poles (14.5423, 5.6082) (14.2605, 5.6873) (13.7909, 5.7961) (13.44, 5.8851) knots 0 0 0 1 2 2 2
  spline S162 degree 2 poles (13.44, 5.8851) (13.1236, 5.9691) (12.6243, 6.2212) (12.4315, 6.4239) knots 0 0 0 1 2 2 2
  spline S163 degree 2 poles (12.4315, 6.4239) (12.2437, 6.6266) (12.0361, 7.1703) (12.0361, 7.5262) knots 0 0 0 1 2 2 2
  spline S164 degree 2 poles (12.0361, 7.5262) (12.0361, 8.2677) (13.1928, 9.2712) (14.0875, 9.2712) knots 0 0 0 1 2 2 2
  spline S165 degree 2 poles (14.0875, 9.2712) (14.6016, 9.2712) (15.5112, 9.0685) (15.9017, 8.8758) knots 0 0 0 1 2 2 2
  line L222 (15.9017, 8.8758) -> (15.9017, 7.9069)
  line L223 (15.9017, 7.9069) -> (15.8424, 7.9069)
  spline S166 degree 2 poles (15.8424, 7.9069) (15.5507, 8.1738) (14.6412, 8.5693) (14.1419, 8.5693) knots 0 0 0 1 2 2 2
  spline S167 degree 2 poles (14.1419, 8.5693) (13.5784, 8.5693) (12.8814, 8.0403) (12.8814, 7.6103) knots 0 0 0 1 2 2 2
  spline S168 degree 2 poles (12.8814, 7.6103) (12.8814, 7.2247) (13.2917, 6.765) (13.6772, 6.6612) knots 0 0 0 1 2 2 2
  spline S169 degree 2 poles (13.6772, 6.6612) (13.9343, 6.592) (14.6807, 6.414) (14.9279, 6.3399) knots 0 0 0 1 2 2 2
  spline S170 degree 2 poles (14.9279, 6.3399) (15.5557, 6.1471) (16.139, 5.371) (16.139, 4.8025) knots 0 0 0 1 2 2 2
  spline S171 degree 2 poles (16.139, 4.8025) (16.139, 4.4416) (15.8473, 3.7496) (15.5853, 3.5074) knots 0 0 0 1 2 2 2
  spline S172 degree 2 poles (15.5853, 3.5074) (15.2937, 3.2404) (14.5522, 2.9537) (13.9936, 2.9537) knots 0 0 0 1 2 2 2
  spline S173 degree 2 poles (18.2893, 2.9735) (17.6615, 2.9735) (16.9546, 3.6903) (16.9546, 4.4664) knots 0 0 0 1 2 2 2
  line L224 (16.9546, 4.4664) -> (16.9546, 7.0023)
  line L225 (16.9546, 7.0023) -> (16.4356, 7.0023)
  line L226 (16.4356, 7.0023) -> (16.4356, 7.6399)
  line L227 (16.4356, 7.6399) -> (16.9546, 7.6399)
  line L228 (16.9546, 7.6399) -> (16.9546, 8.9548)
  line L229 (16.9546, 8.9548) -> (17.7258, 8.9548)
  line L230 (17.7258, 8.9548) -> (17.7258, 7.6399)
  line L231 (17.7258, 7.6399) -> (19.1445, 7.6399)
  line L232 (19.1445, 7.6399) -> (19.1445, 7.0023)
  line L233 (19.1445, 7.0023) -> (17.7258, 7.0023)
  line L234 (17.7258, 7.0023) -> (17.7258, 4.8223)
  spline S174 degree 2 poles (17.7258, 4.8223) (17.7258, 4.4762) (17.7505, 4.0956) (17.8345, 3.9325) knots 0 0 0 1 2 2 2
  spline S175 degree 2 poles (17.8345, 3.9325) (17.9037, 3.7891) (18.2152, 3.6458) (18.4821, 3.6458) knots 0 0 0 1 2 2 2
  spline S176 degree 2 poles (18.4821, 3.6458) (18.6699, 3.6458) (19.0209, 3.7595) (19.1, 3.7941) knots 0 0 0 1 2 2 2
  line L235 (19.1, 3.7941) -> (19.1445, 3.7941)
  line L236 (19.1445, 3.7941) -> (19.1445, 3.102)
  spline S177 degree 2 poles (19.1445, 3.102) (18.927, 3.0427) (18.4821, 2.9735) (18.2893, 2.9735) knots 0 0 0 1 2 2 2
  spline S178 degree 2 poles (22.2637, 3.5469) (22.1698, 3.4777) (21.8534, 3.2305) (21.7051, 3.1564) knots 0 0 0 1 2 2 2
  spline S179 degree 2 poles (21.7051, 3.1564) (21.5024, 3.0476) (21.1218, 2.9339) (20.7758, 2.9339) knots 0 0 0 1 2 2 2
  spline S180 degree 2 poles (20.7758, 2.9339) (20.494, 2.9339) (19.9849, 3.1465) (19.7921, 3.3393) knots 0 0 0 1 2 2 2
  spline S181 degree 2 poles (19.7921, 3.3393) (19.6092, 3.5271) (19.3867, 4.0808) (19.3867, 4.3873) knots 0 0 0 1 2 2 2
  spline S182 degree 2 poles (19.3867, 4.3873) (19.3867, 4.8618) (19.7871, 5.5341) (20.2221, 5.7269) knots 0 0 0 1 2 2 2
  spline S183 degree 2 poles (20.2221, 5.7269) (20.6077, 5.9048) (21.6557, 6.0383) (22.2637, 6.0729) knots 0 0 0 1 2 2 2
  line L237 (22.2637, 6.0729) -> (22.2637, 6.2212)
  spline S184 degree 2 poles (22.2637, 6.2212) (22.2637, 6.4882) (22.1006, 6.8194) (21.9523, 6.9133) knots 0 0 0 1 2 2 2
  spline S185 degree 2 poles (21.9523, 6.9133) (21.804, 7.0072) (21.3789, 7.0665) (21.1515, 7.0665) knots 0 0 0 1 2 2 2
  spline S186 degree 2 poles (21.1515, 7.0665) (20.8845, 7.0665) (20.1628, 6.9083) (19.802, 6.7551) knots 0 0 0 1 2 2 2
  line L238 (19.802, 6.7551) -> (19.7575, 6.7551)
  line L239 (19.7575, 6.7551) -> (19.7575, 7.5411)
  spline S187 degree 2 poles (19.7575, 7.5411) (19.97, 7.6004) (20.7659, 7.7487) (21.1564, 7.7487) knots 0 0 0 1 2 2 2
  spline S188 degree 2 poles (21.1564, 7.7487) (21.631, 7.7487) (22.2785, 7.6004) (22.5356, 7.4076) knots 0 0 0 1 2 2 2
  spline S189 degree 2 poles (22.5356, 7.4076) (22.7877, 7.2198) (23.0349, 6.6216) (23.0349, 6.1916) knots 0 0 0 1 2 2 2
  line L240 (23.0349, 6.1916) -> (23.0349, 3.0625)
  line L241 (23.0349, 3.0625) -> (22.2637, 3.0625)
  line L242 (22.2637, 3.0625) -> (22.2637, 3.5469)
  line L243 (22.2637, 4.1895) -> (22.2637, 5.46)
  spline S190 degree 2 poles (22.2637, 5.46) (21.9869, 5.4352) (21.1515, 5.3512) (20.8895, 5.2721) knots 0 0 0 1 2 2 2
  spline S191 degree 2 poles (20.8895, 5.2721) (20.583, 5.1782) (20.1826, 4.7877) (20.1826, 4.4416) knots 0 0 0 1 2 2 2
  spline S192 degree 2 poles (20.1826, 4.4416) (20.1826, 4.0462) (20.6275, 3.6458) (21.0526, 3.6458) knots 0 0 0 1 2 2 2
  spline S193 degree 2 poles (21.0526, 3.6458) (21.4135, 3.6458) (22.0067, 3.9572) (22.2637, 4.1895) knots 0 0 0 1 2 2 2
  line L244 (27.7112, 3.0625) -> (26.94, 3.0625)
  line L245 (26.94, 3.0625) -> (26.94, 5.6725)
  spline S194 degree 2 poles (26.94, 5.6725) (26.94, 5.9889) (26.8807, 6.5326) (26.7917, 6.6958) knots 0 0 0 1 2 2 2
  spline S195 degree 2 poles (26.7917, 6.6958) (26.6978, 6.8688) (26.3617, 7.0369) (26.075, 7.0369) knots 0 0 0 1 2 2 2
  spline S196 degree 2 poles (26.075, 7.0369) (25.7883, 7.0369) (25.1802, 6.7304) (24.8886, 6.4832) knots 0 0 0 1 2 2 2
  line L246 (24.8886, 6.4832) -> (24.8886, 3.0625)
  line L247 (24.8886, 3.0625) -> (24.1174, 3.0625)
  line L248 (24.1174, 3.0625) -> (24.1174, 7.6399)
  line L249 (24.1174, 7.6399) -> (24.8886, 7.6399)
  line L250 (24.8886, 7.6399) -> (24.8886, 7.1308)
  spline S197 degree 2 poles (24.8886, 7.1308) (25.2346, 7.4422) (25.902, 7.7685) (26.2776, 7.7685) knots 0 0 0 1 2 2 2
  spline S198 degree 2 poles (26.2776, 7.7685) (26.9499, 7.7685) (27.7112, 6.8787) (27.7112, 6.0334) knots 0 0 0 1 2 2 2
  line L251 (27.7112, 6.0334) -> (27.7112, 3.0625)
  line L252 (32.3134, 3.0625) -> (31.5422, 3.0625)
  line L253 (31.5422, 3.0625) -> (31.5422, 3.5271)
  spline S199 degree 2 poles (31.5422, 3.5271) (31.3643, 3.3788) (31.1023, 3.1811) (30.9243, 3.0971) knots 0 0 0 1 2 2 2
  spline S200 degree 2 poles (30.9243, 3.0971) (30.7612, 3.018) (30.4102, 2.9339) (30.1779, 2.9339) knots 0 0 0 1 2 2 2
  spline S201 degree 2 poles (30.1779, 2.9339) (29.8022, 2.9339) (29.1695, 3.2454) (28.947, 3.5469) knots 0 0 0 1 2 2 2
  spline S202 degree 2 poles (28.947, 3.5469) (28.7246, 3.8484) (28.4774, 4.7382) (28.4774, 5.3166) knots 0 0 0 1 2 2 2
  spline S203 degree 2 poles (28.4774, 5.3166) (28.4774, 5.9197) (28.7888, 6.7996) (29.0607, 7.1308) knots 0 0 0 1 2 2 2
  spline S204 degree 2 poles (29.0607, 7.1308) (29.3128, 7.4274) (30.0197, 7.7685) (30.4102, 7.7685) knots 0 0 0 1 2 2 2
  spline S205 degree 2 poles (30.4102, 7.7685) (30.7513, 7.7685) (31.2605, 7.6152) (31.5422, 7.457) knots 0 0 0 1 2 2 2
  line L254 (31.5422, 7.457) -> (31.5422, 9.4343)
  line L255 (31.5422, 9.4343) -> (32.3134, 9.4343)
  line L256 (32.3134, 9.4343) -> (32.3134, 3.0625)
  line L257 (31.5422, 4.1747) -> (31.5422, 6.8194)
  spline S206 degree 2 poles (31.5422, 6.8194) (31.2555, 6.9578) (30.8007, 7.0616) (30.5387, 7.0616) knots 0 0 0 1 2 2 2
  spline S207 degree 2 poles (30.5387, 7.0616) (29.9456, 7.0616) (29.2733, 6.1718) (29.2733, 5.3314) knots 0 0 0 1 2 2 2
  spline S208 degree 2 poles (29.2733, 5.3314) (29.2733, 4.5207) (29.7874, 3.6655) (30.3558, 3.6655) knots 0 0 0 1 2 2 2
  spline S209 degree 2 poles (30.3558, 3.6655) (30.6574, 3.6655) (31.2704, 3.9424) (31.5422, 4.1747) knots 0 0 0 1 2 2 2
  spline S210 degree 2 poles (37.2665, 5.4253) (37.2665, 4.3032) (36.179, 2.9339) (35.3584, 2.9339) knots 0 0 0 1 2 2 2
  spline S211 degree 2 poles (35.3584, 2.9339) (34.9877, 2.9339) (34.4588, 3.1168) (34.2017, 3.275) knots 0 0 0 1 2 2 2
  line L258 (34.2017, 3.275) -> (34.1523, 3.0625)
  line L259 (34.1523, 3.0625) -> (33.4306, 3.0625)
  line L260 (33.4306, 3.0625) -> (33.4306, 9.4343)
  line L261 (33.4306, 9.4343) -> (34.2017, 9.4343)
  line L262 (34.2017, 9.4343) -> (34.2017, 7.1604)
  spline S212 degree 2 poles (34.2017, 7.1604) (34.4934, 7.4224) (35.1706, 7.7685) (35.6007, 7.7685) knots 0 0 0 1 2 2 2
  spline S213 degree 2 poles (35.6007, 7.7685) (36.3768, 7.7685) (37.2665, 6.5277) (37.2665, 5.4253) knots 0 0 0 1 2 2 2
  spline S214 degree 2 poles (36.4707, 5.366) (36.4707, 6.1866) (35.9714, 7.0369) (35.4178, 7.0369) knots 0 0 0 1 2 2 2
  spline S215 degree 2 poles (35.4178, 7.0369) (35.1063, 7.0369) (34.4637, 6.7403) (34.2017, 6.5129) knots 0 0 0 1 2 2 2
  line L263 (34.2017, 6.5129) -> (34.2017, 3.888)
  spline S216 degree 2 poles (34.2017, 3.888) (34.4934, 3.7446) (34.9432, 3.626) (35.2101, 3.626) knots 0 0 0 1 2 2 2
  spline S217 degree 2 poles (35.2101, 3.626) (35.7984, 3.626) (36.4707, 4.4614) (36.4707, 5.366) knots 0 0 0 1 2 2 2
  line L264 (41.6611, 7.6399) -> (39.1994, 1.3768)
  line L265 (39.1994, 1.3768) -> (38.3738, 1.3768)
  line L266 (38.3738, 1.3768) -> (39.1944, 3.2849)
  line L267 (39.1944, 3.2849) -> (37.5335, 7.6399)
  line L268 (37.5335, 7.6399) -> (38.364, 7.6399)
  line L269 (38.364, 7.6399) -> (39.6146, 4.2488)
  line L270 (39.6146, 4.2488) -> (40.8603, 7.6399)
  line L271 (40.8603, 7.6399) -> (41.6611, 7.6399)
  line L272 (16.118, -11.8179) -> (12.3562, -11.8179)
  line L273 (12.3562, -11.8179) -> (12.3562, -10.9528)
  spline S218 degree 2 poles (12.3562, -10.9528) (12.7616, -10.5722) (13.4833, -9.8653) (13.8293, -9.4847) knots 0 0 0 1 2 2 2
  spline S219 degree 2 poles (13.8293, -9.4847) (14.5263, -8.7185) (15.0355, -7.799) (15.0355, -7.3096) knots 0 0 0 1 2 2 2
  spline S220 degree 2 poles (15.0355, -7.3096) (15.0355, -7.0526) (14.8773, -6.667) (14.7339, -6.5434) knots 0 0 0 1 2 2 2
  spline S221 degree 2 poles (14.7339, -6.5434) (14.5906, -6.4198) (14.2149, -6.2962) (13.9875, -6.2962) knots 0 0 0 1 2 2 2
  spline S222 degree 2 poles (13.9875, -6.2962) (13.77, -6.2962) (13.3251, -6.405) (13.1224, -6.489) knots 0 0 0 1 2 2 2
  spline S223 degree 2 poles (13.1224, -6.489) (12.9494, -6.5582) (12.6281, -6.756) (12.5292, -6.8252) knots 0 0 0 1 2 2 2
  line L274 (12.5292, -6.8252) -> (12.4847, -6.8252)
  line L275 (12.4847, -6.8252) -> (12.4847, -5.9552)
  spline S224 degree 2 poles (12.4847, -5.9552) (12.7368, -5.8316) (13.6415, -5.5894) (14.0468, -5.5894) knots 0 0 0 1 2 2 2
  spline S225 degree 2 poles (14.0468, -5.5894) (14.902, -5.5894) (15.8659, -6.494) (15.8659, -7.2651) knots 0 0 0 1 2 2 2
  spline S226 degree 2 poles (15.8659, -7.2651) (15.8659, -7.626) (15.6979, -8.2291) (15.5496, -8.4861) knots 0 0 0 1 2 2 2
  spline S227 degree 2 poles (15.5496, -8.4861) (15.4013, -8.7531) (14.9712, -9.277) (14.7339, -9.5292) knots 0 0 0 1 2 2 2
  spline S228 degree 2 poles (14.7339, -9.5292) (14.3484, -9.9493) (13.4042, -10.849) (13.1224, -11.111) knots 0 0 0 1 2 2 2
  line L276 (13.1224, -11.111) -> (16.118, -11.111)
  line L277 (16.118, -11.111) -> (16.118, -11.8179)
  line L278 (20.8586, -9.7219) -> (20.132, -9.7219)
  line L279 (20.132, -9.7219) -> (20.132, -11.8179)
  line L280 (20.132, -11.8179) -> (19.346, -11.8179)
  line L281 (19.346, -11.8179) -> (19.346, -9.7219)
  line L282 (19.346, -9.7219) -> (16.6519, -9.7219)
  line L283 (16.6519, -9.7219) -> (16.6519, -8.8618)
  line L284 (16.6519, -8.8618) -> (19.3806, -5.7179)
  line L285 (19.3806, -5.7179) -> (20.132, -5.7179)
  line L286 (20.132, -5.7179) -> (20.132, -9.0645)
  line L287 (20.132, -9.0645) -> (20.8586, -9.0645)
  line L288 (20.8586, -9.0645) -> (20.8586, -9.7219)
  line L289 (19.346, -9.0645) -> (19.346, -6.6818)
  line L290 (19.346, -6.6818) -> (17.2945, -9.0645)
  line L291 (17.2945, -9.0645) -> (19.346, -9.0645)
  line L292 (26.1084, -5.7179) -> (24.0075, -11.8179)
  line L293 (24.0075, -11.8179) -> (23.1326, -11.8179)
  line L294 (23.1326, -11.8179) -> (21.0317, -5.7179)
  line L295 (21.0317, -5.7179) -> (21.9017, -5.7179)
  line L296 (21.9017, -5.7179) -> (23.5923, -10.7847)
  line L297 (23.5923, -10.7847) -> (25.2829, -5.7179)
  line L298 (25.2829, -5.7179) -> (26.1084, -5.7179)
  spline S229 degree 2 poles (31.0715, -11.9217) (30.5969, -11.9217) (29.8109, -11.63) (29.5291, -11.3334) knots 0 0 0 1 2 2 2
  spline S230 degree 2 poles (29.5291, -11.3334) (29.2474, -11.0418) (28.936, -10.1421) (28.936, -9.539) knots 0 0 0 1 2 2 2
  spline S231 degree 2 poles (28.936, -9.539) (28.936, -8.936) (29.2573, -8.0561) (29.5291, -7.7595) knots 0 0 0 1 2 2 2
  spline S232 degree 2 poles (29.5291, -7.7595) (29.801, -7.4579) (30.6068, -7.1366) (31.0715, -7.1366) knots 0 0 0 1 2 2 2
  spline S233 degree 2 poles (31.0715, -7.1366) (31.4471, -7.1366) (32.1491, -7.3492) (32.421, -7.4876) knots 0 0 0 1 2 2 2
  line L299 (32.421, -7.4876) -> (32.421, -8.3527)
  line L300 (32.421, -8.3527) -> (32.3765, -8.3527)
  spline S234 degree 2 poles (32.3765, -8.3527) (32.2924, -8.2834) (32.0354, -8.1055) (31.8525, -8.0116) knots 0 0 0 1 2 2 2
  spline S235 degree 2 poles (31.8525, -8.0116) (31.6894, -7.9325) (31.2544, -7.8089) (31.0566, -7.8089) knots 0 0 0 1 2 2 2
  spline S236 degree 2 poles (31.0566, -7.8089) (30.4585, -7.8089) (29.7318, -8.7135) (29.7318, -9.539) knots 0 0 0 1 2 2 2
  spline S237 degree 2 poles (29.7318, -9.539) (29.7318, -10.3448) (30.4338, -11.2494) (31.0566, -11.2494) knots 0 0 0 1 2 2 2
  spline S238 degree 2 poles (31.0566, -11.2494) (31.4323, -11.2494) (32.1145, -10.938) (32.3765, -10.6958) knots 0 0 0 1 2 2 2
  line L301 (32.3765, -10.6958) -> (32.421, -10.6958)
  line L302 (32.421, -10.6958) -> (32.421, -11.5608)
  spline S239 degree 2 poles (32.421, -11.5608) (32.3073, -11.6152) (31.9612, -11.7685) (31.8228, -11.8031) knots 0 0 0 1 2 2 2